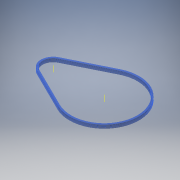
# Autodesk Inventor part: Roller Chain
Saved by Autodesk Inventor 2016 (Build 200138000, 138)
## iProperties
Created: 2016-04-25
Part Number: Roller Chain
Material: Generic
Document SubType Name: Modeling
Designer: Henrik Samuelsson
Density: 1 g/cm^3
Appearance: Clear - Blue
CustomPartVersion: 1
Author: Henrik Samuelsson
Autodesk Inventor part; units mm, degrees
ref_plane "Work Plane2" through (-271.2696, 0, 0) normal (-1, 0, 0) x (0, 0, 1)
ref_plane "Work Plane3" through (127, 0, 0) normal (-0.9043554, -0.4267802, 0) x (0, 0, 1)
sketch "Path" plane through (0, 0, 0) normal (0, 0, 1) x (1, 0, 0)
  arc A0 (-310.5685, 79.5561) -> (-310.5685, -79.5561) centre (-271.2696, 0) ccw
  arc A1 (9.5802, -237.7025) -> (9.5802, 237.7025) centre (127, 0) ccw
  line L0 (9.5802, -237.7025) -> (-310.5685, -79.5561)
  line L1 (-310.5685, 79.5561) -> (9.5802, 237.7025)
  dimension "d31" = 13.5
  constraints: 4 end point, 4 point on circle, 2 centre point
ref_plane "Section Plane" through (-310.5685, -79.5561, 0) normal (0.8965764, -0.4428891, 0) x (0, 0, 1)
sketch "Section Sketch" plane through (-310.5685, -79.5561, 0) normal (0.8965764, -0.4428891, 0) x (0, 0, 1)
  line L0 (-13.35, -2.235) -> (13.35, -2.235)
  line L1 (13.35, -2.235) -> (13.35, 2.235)
  line L2 (13.35, 2.235) -> (-13.35, 2.235)
  line L3 (-13.35, 2.235) -> (-13.35, -2.235)
  line L4 (-7.94, -5.715) -> (7.94, -5.715)
  line L5 (7.94, -5.715) -> (7.94, 5.715)
  line L6 (7.94, 5.715) -> (-7.94, 5.715)
  line L7 (-7.94, 5.715) -> (-7.94, -5.715)
  line L8 (-7.94, 0) -> (7.94, 0) construction
  line L9 (-13.782, -6.75) -> (-7.94, -6.75)
  line L10 (-7.94, -6.75) -> (-7.94, 6.75)
  line L11 (-7.94, 6.75) -> (-13.782, 6.75)
  line L12 (-13.782, 6.75) -> (-13.782, -6.75)
  line L13 (7.94, -6.75) -> (13.782, -6.75)
  line L14 (13.782, -6.75) -> (13.782, 6.75)
  line L15 (13.782, 6.75) -> (7.94, 6.75)
  line L16 (7.94, 6.75) -> (7.94, -6.75)
  line L17 (-13.35, 0) -> (13.35, 0) construction
  point P0 (0, 0)
  point P1 (0, 0)
  dimension "d21" = 4.47
  dimension "d22" = 11.43
  dimension "d23" = 15.88
  dimension "d24" = 5.842
  dimension "d31" = 13.5
  dimension "d32" = 26.7
  constraints: 36 end point, 8 midpoint, 8 parallel, 4 horizontal, 4 perpendicular, 3 collinear, 1 coincident, 1 other
  measures "d21" distance between parallel lines of L2 L0
  measures "d22" distance between parallel lines of L6 L4
  measures "d23" distance between parallel lines of L5 L7
  measures "d24" distance between parallel lines of L12 L10
  measures "d31" distance between parallel lines of L11 L9
  measures "d32" distance between parallel lines of L1 L3
sweep "Solid" add profiles "Section Sketch" path "Path"
pattern_of_one "Strand Pattern"
equation "\"d21\" = da_d2"
equation "\"d22\" = da_d1"
equation "\"d23\" = da_b1"
equation "\"d24\" = da_t1 + da_t2"
equation "\"d30\" = da_pt"
equation "\"da_p\" = 29.21"
equation "\"da_b1\" = 15.88"
equation "\"da_h2\" = 13.5"
equation "\"da_h3\" = 13.5"
equation "\"da_d1\" = 11.43"
equation "\"da_d2\" = 4.47"
equation "\"da_pt\" = 25"
equation "\"da_b\" = 26.7"
equation "\"da_t1\" = 2.921"
equation "\"da_t2\" = 2.921"
body "Solid1"
